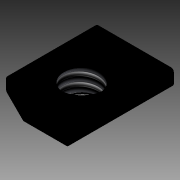
# Autodesk Inventor part: 3204
Saved by Autodesk Inventor 2014 SP2 (Build 180246200, 246)
## iProperties
Created: 2019-11-08
Part Number: 3204
Material: Generic
Catalog Web Link: www.cadenas.de
Description: 3205, 3204, 3206, 3871, 3873, 8901, 8901-36, 3201, 3202, 3203, 3866, 3703, 3868, 8900, 8900-36-Slide-In T-Nuts
Vendor: 8020
Document SubType Name: Modeling
Designer: psadmin
Manufacturer: 8020
Mass: 0.427329 g
Surface Area: 4.41997 cm^2
Volume: 0.427329 cm^3
Density: 1 g/cm^3
Appearance: PSOLRGB-0-0-0
Category: PARTsolutions
Company: 8020
Title: 3204
Author: Cadenas PARTsolutions
Comments: Slide-In T-Nuts
PSOL_IDENT_0: {$CADENAS_DATA\23d-libs\8020\inch\fastening_options\3205.prj},236 {VTYP=3D},{NB=3204},{LINA=3204},{N
PSOL_IDENT_1: N=3205, 3204, 3206, 3871, 3873, 8901, 8901-36, 3201, 3202, 3203, 3866, 3703, 3868, 8900, 8900-36},{D
PSOL_IDENT_2: ATE=01.10.2019 06:04:21},{GEOMDATE=29.05.2019 18:10:24},{VERSION=},{LINEID=30},{WBVAR=},{WBNUMERIC=}
PSOL_IDENT_3: {NB=3204},{LINA=3204},{KT=DUMMY},{PN=3204},{MAT=1215 Carbon Steel},{FIN=Black Zinc},{A=0.171},{B=.
PSOL_IDENT_4: 200},{B1=0.200},{C=.490},{C1=0.490},{D=0.431},{E=1/4-20},{E1=0.25000},{TT=UNC},{W=.010},{COL=0.00,0.
PSOL_IDENT_5: 00,0.00,0.00},{NO=2}
NN: 3205, 3204, 3206, 3871, 3873, 8901, 8901-36, 3201, 3202, 3203, 3866, 3703, 3868, 8900, 8900-36
NT: Slide-In T-Nuts
NB: 3204
NBSYN: $PN.
LINA: 3204
PN: 3204
MAT: 1215 Carbon Steel
FIN: Black Zinc
A: 0.171
B: .200
C: .490
D: 0.431
E: 1/4-20
W: .010
SUPPLIER: 8020
ARTICLENO: 3204
BOMINFO: 3204
CREATOR: CADENAS GmbH
Autodesk Inventor part; units mm, degrees
sketch "Sketch_1" plane through (0, 0, -7.366) normal (0, 0, 1) x (1, 0, 0)
  line L0 (-5.4737, 3.9624) -> (-5.4737, 2.5467)
  arc A0 (-5.4737, 2.5467) -> (-5.3621, 2.2773) centre (-5.0927, 2.5467) ccw
  line L1 (-5.3621, 2.2773) -> (-3.1964, 0.1116)
  arc A1 (-3.1964, 0.1116) -> (-2.927, 0) centre (-2.927, 0.381) ccw
  line L2 (-2.927, 0) -> (2.927, 0)
  arc A2 (2.927, 0) -> (3.1964, 0.1116) centre (2.927, 0.381) ccw
  line L3 (3.1964, 0.1116) -> (5.3621, 2.2773)
  arc A3 (5.3621, 2.2773) -> (5.4737, 2.5467) centre (5.0927, 2.5467) ccw
  line L4 (5.4737, 2.5467) -> (5.4737, 3.9624)
  arc A4 (5.4737, 3.9624) -> (5.0927, 4.3434) centre (5.0927, 3.9624) ccw
  line L5 (5.0927, 4.3434) -> (-5.0927, 4.3434)
  arc A5 (-5.0927, 4.3434) -> (-5.4737, 3.9624) centre (-5.0927, 3.9624) ccw
  constraints: 12 end point, 12 point on circle, 6 centre point
extrude "Extrusion1" add sketch "Sketch_1" along normal blind 12.446
sketch "Sketch_3" plane through (0, 0, 0) normal (0, 0, 1) x (1, 0, 0)
  line L0 (0, 0) -> (0, 4.3434)
  line L1 (0, 4.3434) -> (3.175, 4.3434)
  line L2 (3.175, 4.3434) -> (2.4879, 3.6563)
  line L3 (2.4879, 3.6563) -> (2.4879, 0.6871)
  line L4 (2.4879, 0.6871) -> (3.175, 0)
  line L5 (3.175, 0) -> (0, 0)
  line L6 (0, 0) -> (0, 4.3434)
  constraints: 14 end point
revolve "Revolution1" cut sketch "Sketch_3" angle 360 about axis through (0, 0, 0) along (0, -1, 0)
thread "Thread1" size "1/4-20 UNC" class "2B" standard "ANSI Unified Screw Threads" full length
ref_plane "tnut_XY" through (0, 4.3434, 0) normal (0, 1, 0) x (1, 0, 0)
ref_plane "tnut_YZ" through (0, 4.3434, 0) normal (1, 0, 0) x (0, 0, -1)
ref_plane "tnut_ZX" through (0, 4.3434, 0) normal (0, 0, -1) x (0, 1, 0)
body "Solid1"
